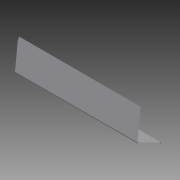
# Autodesk Inventor part: stopper plate
Saved by Autodesk Inventor 2015 SP1 (Build 190203100, 203)
## iProperties
Created: 2015-02-08
Part Number: stopper plate
Material: Generic
Document SubType Name: Modeling
Designer: Admin
Density: 1 g/cm^3
Appearance: Default
Author: Admin
Autodesk Inventor part; units mm, degrees
ref_plane "YZ Plane" through (0, 0, 0) normal (1, 0, 0) x (0, 1, 0)
ref_plane "XZ Plane" through (0, 0, 0) normal (0, 1, 0) x (-1, 0, 0)
ref_plane "XY Plane" through (0, 0, 0) normal (0, 0, 1) x (1, 0, 0)
sketch "Sketch1" plane through (0, 0, 0) normal (1, 0, 0) x (0, 1, 0)
  line L0 (0, 0) -> (1.5875, 0)
  line L1 (1.5875, 0) -> (1.5875, -50.8)
  line L2 (1.5875, -50.8) -> (0, -50.8)
  line L3 (0, -50.8) -> (0, 0)
  line L4 (1.5875, 0) -> (45.5816, -25.4)
  line L5 (45.5816, -25.4) -> (44.7878, -26.7748)
  line L6 (44.7878, -26.7748) -> (0.7938, -1.3748)
  line L7 (0.7938, -1.3748) -> (1.5875, 0)
  line L8 (1.5875, 0) -> (52.3875, 0) construction
  dimension "d0" = 1.5875
  dimension "d1" = 50.8
  dimension "d2" = 50.8
  dimension "d3" = 30
  dimension "d4" = 1.5875
  constraints: 18 end point, 4 parallel, 2 horizontal, 2 perpendicular, 1 equal length
  measures "d0" distance of L1.end L2.end
  measures "d1" distance of L0.end L1.end
  measures "d2" distance of L0.end L4.end
  measures "d3" angle of L4 L8
  measures "d4" distance of L4.end L5.end
extrude "Extrusion1" add sketch "Sketch1" along normal blind 304.8
sketch "Sketch2" plane through (0, 0, -50.8) normal (0, -1, 0) x (1, 0, 0)
  line L0 (0, 0) -> (304.8, 0) projected
  line L1 (304.8, 50.8) -> (304.8, 0) projected
  point P0 (177.8, 28.575)
  point P1 (127, 28.575)
  dimension "d7" = 28.575
  dimension "d8" = 28.575
  dimension "d9" = 127
  dimension "d10" = 177.8
  measures "d7" distance from line of L0 point (177.8, 28.575)
  measures "d8" distance from line of L0 point (127, 28.575)
  measures "d9" distance from line of L1 point (177.8, 28.575)
  measures "d10" distance from line of L1 point (127, 28.575)
hole "Hole1" at (177.8, 0, -22.225) at (127, 0, -22.225) direction (0, 1, 0) diameter 6.35 depth 6.35 tip angle 118
sketch "Sketch5" plane through (0, 1.5875, -1.8331) normal (0, 1, 0) x (1, 0, 0)
  line L0 (0, 48.9669) -> (304.8, 48.9669) projected
  line L1 (0, 48.9669) -> (101.6, 48.9669)
  line L2 (101.6, 48.9669) -> (101.6, 23.5669)
  line L3 (101.6, 23.5669) -> (0, 23.5669)
  line L4 (0, 23.5669) -> (0, 48.9669)
  line L5 (304.8, 48.9669) -> (203.2, 48.9669)
  line L6 (203.2, 48.9669) -> (203.2, 23.5669)
  line L7 (203.2, 23.5669) -> (304.8, 23.5669)
  line L8 (304.8, 23.5669) -> (304.8, 48.9669)
  line L9 (203.2, 48.9669) -> (177.8, 48.9669)
  line L10 (177.8, 48.9669) -> (203.2, 23.5669)
  line L11 (101.6, 48.9669) -> (127, 48.9669)
  line L12 (0, 48.9669) -> (304.8, 48.9669) projected
  line L13 (127, 48.9669) -> (101.6, 23.5669)
  point P0 (0, -1.8331)
  dimension "d28" = 101.6
  dimension "d29" = 25.4
  dimension "d30" = 101.6
  dimension "d31" = 25.4
  dimension "d32" = 25.4
  dimension "d33" = 25.4
  constraints: 24 end point, 4 parallel, 2 horizontal, 2 perpendicular, 2 point on line
  measures "d28" distance of L2.end L3.end
  measures "d29" distance of L1.end L2.end
  measures "d30" distance of L7.end L6.end
  measures "d31" distance of L6.end L5.end
  measures "d32" distance of L5.end L9.end
  measures "d33" distance of L1.end L11.end
extrude "Extrusion4" cut sketch "Sketch5" against normal blind 6.35
body "Solid1"
